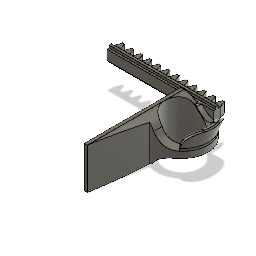
920-002_DynamicFinger (Autodesk Fusion 360 design; units mm, degrees)
Autodesk Fusion 360 part; units mm, degrees
sketch "Sketch1" plane through (0, 0, 0) normal (0, 1, 0) x (1, 0, 0)
  line L0 (0, 0) -> (-12, 0) construction
  line L1 (0.72794, -2) -> (-0.72794, 2)
  line L2 (-1.374447, -2) -> (-1.374447, 4.5) construction
  line L3 (-3.476834, -2) -> (-2.020953, 2)
  line L4 (-2.020953, 2) -> (-0.72794, 2)
  line L5 (0.72794, -2) -> (0.72794, -6)
  line L6 (0.72794, -6) -> (-63.952493, -6)
  line L7 (-4.769847, -2) -> (-6.225728, 2)
  line L8 (-7.51874, 2) -> (-6.225728, 2)
  line L9 (-8.974621, -2) -> (-7.51874, 2)
  line L10 (-10.267634, -2) -> (-11.723515, 2)
  line L11 (-13.016527, 2) -> (-11.723515, 2)
  line L12 (-14.472408, -2) -> (-13.016527, 2)
  line L13 (-15.765421, -2) -> (-17.221302, 2)
  line L14 (-18.514315, 2) -> (-17.221302, 2)
  line L15 (-19.970195, -2) -> (-18.514315, 2)
  line L16 (-21.263208, -2) -> (-22.719089, 2)
  line L17 (-24.012102, 2) -> (-22.719089, 2)
  line L18 (-25.467983, -2) -> (-24.012102, 2)
  line L19 (-26.760995, -2) -> (-28.216876, 2)
  line L20 (-29.509889, 2) -> (-28.216876, 2)
  line L21 (-30.96577, -2) -> (-29.509889, 2)
  line L22 (-32.258782, -2) -> (-33.714663, 2)
  line L23 (-35.007676, 2) -> (-33.714663, 2)
  line L24 (-36.463557, -2) -> (-35.007676, 2)
  line L25 (-37.75657, -2) -> (-39.21245, 2)
  line L26 (-40.505463, 2) -> (-39.21245, 2)
  line L27 (-41.961344, -2) -> (-40.505463, 2)
  line L28 (-43.254357, -2) -> (-44.710238, 2)
  line L29 (-46.00325, 2) -> (-44.710238, 2)
  line L30 (-47.459131, -2) -> (-46.00325, 2)
  line L31 (-48.752144, -2) -> (-50.208025, 2)
  line L32 (-51.501037, 2) -> (-50.208025, 2)
  line L33 (-52.956918, -2) -> (-51.501037, 2)
  line L34 (-54.249931, -2) -> (-55.705812, 2)
  line L35 (-56.998825, 2) -> (-55.705812, 2)
  line L36 (-58.454705, -2) -> (-56.998825, 2)
  line L37 (-59.747718, -2) -> (-61.203599, 2)
  line L38 (-62.496612, 2) -> (-61.203599, 2)
  line L39 (-63.952493, -2) -> (-62.496612, 2)
  line L40 (-63.952493, -2) -> (-63.952493, -6)
  line L41 (-59.747718, -2) -> (-58.454705, -2)
  line L42 (-54.249931, -2) -> (-52.956918, -2)
  line L43 (-48.752144, -2) -> (-47.459131, -2)
  line L44 (-43.254357, -2) -> (-41.961344, -2)
  line L45 (-37.75657, -2) -> (-36.463557, -2)
  line L46 (-32.258782, -2) -> (-30.96577, -2)
  line L47 (-26.760995, -2) -> (-25.467983, -2)
  line L48 (-21.263208, -2) -> (-19.970195, -2)
  line L49 (-15.765421, -2) -> (-14.472408, -2)
  line L50 (0.72794, -2) -> (-4.769847, -2) construction
  line L51 (-8.974621, -2) -> (-10.267634, -2) construction
  line L52 (-10.267634, -2) -> (-8.974621, -2)
  line L53 (-4.769847, -2) -> (-3.476834, -2)
  point P0 (-2.748894, 0)
  dimension "d3" = 70
  dimension "d4" = 2.748894
  dimension "d5" = 2
  dimension "d8" = -5.497787
  dimension "d9" = 0
  dimension "d10" = 4
  constraint coincident L0.start origin
  constraint horizontal L0
  constraint horizontal L50
  constraint midpoint L0.start L1
  constraint perpendicular L2 L50
  constraint perpendicular L5 L50
  constraint perpendicular L5 L6
  constraint vertical L40
  constraint collinear L41 L42
  constraint collinear L42 L43
  constraint collinear L43 L44
  constraint collinear L44 L45
  constraint collinear L45 L46
  constraint collinear L46 L47
  constraint collinear L47 L48
  constraint collinear L48 L49
  constraint collinear L49 L52
  constraint collinear L50 L51
  constraint collinear L52 L53
  measures "d3" angle of L1 L50
  measures "d5" distance of L0 L4
extrude "Extrude1" add sketch "Sketch1" along normal blind 6 contours L1 L3 L4 L5 L6 L7 L8 L9 L10 L11 L12 L13 L14 L15 L16 L17 L18 L19 L20 L21 L22 L23 L24 L25 L26 L27 L28 L29 L30 L31 L32 L33 L34 L35 L36 L37 L38 L39 L40 L41 L42 L43 L44 L45 L46 L47 L48 L49 L52 L53 picked at (-31.827778, -4.666667)
sketch "Sketch3" plane through (0.72794, 0, 0) normal (1, 0, 0) x (0, 0, -1)
  line L0 (-6, 0) -> (-2, 0)
  line L1 (-2, 0) -> (-2, 6)
  line L2 (-2, 6) -> (-6, 6)
  line L3 (-6, 6) -> (-6, 0)
  line L4 (-4.75, 6) -> (-4.75, 7.5)
  line L5 (-4.75, 7.5) -> (-3.25, 7.5)
  line L6 (-3.25, 7.5) -> (-3.25, 6)
  line L7 (-4, 6) -> (-4, 0) construction
  line L8 (-4, 6) -> (-4, 7.5) construction
  line L9 (-4, 3) -> (-2.683417, 3) construction
  line L10 (-4.75, 0) -> (-4.75, -1.5)
  line L11 (-4.75, -1.5) -> (-3.25, -1.5)
  line L12 (-3.25, -1.5) -> (-3.25, 0)
  dimension "d15" = 1.5
  dimension "d16" = 1.5
  constraint coincident L2 L4.start
  constraint perpendicular L2 L4
  constraint perpendicular L4 L5
  constraint coincident L2 L6.end
  constraint midpoint L2 L7.start
  constraint midpoint L0 L7.end
  constraint midpoint L5 L8.end
  constraint vertical L8
  constraint vertical L6
  constraint midpoint L7 L9.start
  constraint perpendicular L7 L9
  constraint symmetric L4.start L9 L10.start
  constraint symmetric L4.end L9 L10.end
  constraint symmetric L5.end L9 L11.end
  constraint symmetric L6.end L9 L12.end
  measures "d15" distance of L4.end L5.end
  measures "d16" distance of L4.start L4.end
extrude "Extrude3" add sketch "Sketch3" against normal blind 64.68 contours L0 L10 L11 L12 | L2 L4 L5 L6 picked at (-3.75, -1) picked at (-3.75, 7)
ref_plane "WorkPlane1" through (-18.27206, 3, 4) normal (1, 0, 0) x (0, 0, -1)
ref_plane "WorkPlane2" through (-31.612276, -3.257, 2) normal (0, -1, 0) x (-1, 0, 0)
sketch "Sketch4" plane through (0, 0, 6) normal (0, 0, 1) x (1, 0, 0)
  line L0 (-63.952493, 0) -> (0.72794, 0)
  line L1 (0.72794, 0) -> (0.72794, 6)
  line L2 (0.72794, 6) -> (-63.952493, 6)
  line L3 (-63.952493, 6) -> (-63.952493, 0)
  line L4 (7.195984, -3.257) -> (-70.420536, -3.257) construction
  line L5 (-18.27206, 24.190027) -> (-18.27206, -18.190027) construction
  line L6 (-18.27206, 9.243) -> (-16.27206, 9.243)
  line L7 (-16.27206, 9.243) -> (-16.27206, -15.757)
  line L8 (-16.27206, -15.757) -> (-18.27206, -15.757)
  line L9 (-18.27206, -15.757) -> (-18.27206, 9.243)
  line L10 (-18.27206, 9.243) -> (-16.27206, -15.757) construction
  line L11 (-16.27206, 9.243) -> (-18.27206, -15.757) construction
  point P0 (-17.27206, -3.257)
  dimension "d21" = 25
  dimension "d22" = 2
  constraint perpendicular L6 L7
  constraint parallel L6 L8
  constraint parallel L7 L9
  constraint horizontal L6
extrude "Extrude4" add sketch "Sketch4" along normal blind 59.5 contours L0 L2 L7 L9 | L0 L7 L8 L9 | L2 L6 L7 L9 picked at (-16.938726, 4) picked at (-16.938726, -10.504667) picked at (-17.605393, 8.162)
sketch "Sketch5" plane through (0, 9.243, 0) normal (0, 1, 0) x (-1, 0, 0)
  line L0 (16.27206, 6) -> (18.27206, 6)
  line L1 (18.27206, 6) -> (18.27206, 65.5)
  line L2 (18.27206, 65.5) -> (16.27206, 65.5)
  line L3 (16.27206, 65.5) -> (16.27206, 6)
  line L4 (-0.72794, 6) -> (16.27206, 6)
  line L5 (16.27206, 65.5) -> (6.27206, 6)
  line L6 (6.27206, 6) -> (16.27206, 6)
  line L7 (16.27206, 6) -> (16.27206, 65.5)
  dimension "d25" = 10
extrude "Extrude5" add sketch "Sketch5" against normal blind 25 contours L3 L4 L5 L6 L7 picked at (12.938726, 25.833333)
sketch "Sketch6" plane through (0, 9.243, 0) normal (0, 1, 0) x (-1, 0, 0)
  line L0 (6.27206, 6) -> (18.27206, 6)
  line L1 (18.27206, 6) -> (18.27206, 65.5)
  line L2 (18.27206, 65.5) -> (16.27206, 65.5)
  line L3 (16.27206, 65.5) -> (6.27206, 6)
  line L4 (16.27206, 65.5) -> (16.27206, -17.848583) construction
  circle A0 centre (5.77206, 18.5) radius 10.5
  circle A1 centre (5.77206, 18.5) radius 15.5
  line L5 (5.77206, 18.5) -> (5.77206, 8) construction
  line L6 (6.27206, 6) -> (-0.72794, 6)
  line L7 (16.27206, 65.5) -> (6.27206, 6)
  line L8 (-0.72794, 6) -> (-0.72794, 4.75)
  line L9 (-0.72794, 4.75) -> (-0.72794, 3.25)
  line L10 (-0.72794, 6) -> (6.27206, 6)
  dimension "d28" = 21
  dimension "d29" = 5
  dimension "d30" = 2
  constraint perpendicular L0 L4
  constraint tangent L4 A0
  measures "d28" diameter of A0
extrude "Extrude6" add sketch "Sketch6" against normal blind 25 contours L3 A0 A1 L6 L7 L8 L9 L10 picked at (-1.91992, 7.664105)
sketch "Sketch7" plane through (0, 9.243, 0) normal (0, 1, 0) x (-1, 0, 0)
  line L0 (9.989032, 28.115984) -> (6.613875, 8.0338)
  arc A0 (9.989032, 28.115984) -> (6.613875, 8.0338) centre (5.77206, 18.5) ccw
  arc A1 (10.835048, 33.149783) -> (-0.72794, 4.428753) centre (5.77206, 18.5) ccw
  line L1 (-0.72794, 4.428753) -> (-0.72794, 6)
  line L2 (-0.72794, 6) -> (18.27206, 6)
  line L3 (18.27206, 6) -> (18.27206, 65.5)
  line L4 (18.27206, 65.5) -> (16.27206, 65.5)
  line L5 (16.27206, 65.5) -> (10.835048, 33.149783)
  circle A2 centre (5.77206, 18.5) radius 10.5
  line L6 (-0.72794, 6) -> (-3.393092, 6)
  constraint concentric A0 A2
  constraint perpendicular L1 L6
extrude "Extrude7" cut sketch "Sketch7" against normal through all contours L0 A2 | A1 L1 L6 picked at (9.219892, 15.192215) picked at (-1.035493, 5.107205)
sketch "Sketch8" plane through (0, 0, 0) normal (0, -1, 0) x (1, 0, 0)
  line L0 (-63.95206, 4.75) -> (0.72794, 4.75)
  line L1 (0.72794, 4.75) -> (0.72794, 6)
  line L2 (0.72794, 6) -> (-18.27206, 6)
  line L3 (-18.27206, 6) -> (-63.952493, 6)
  line L4 (-63.952493, 6) -> (-63.952493, 2)
  line L5 (-63.952493, 2) -> (-62.496612, -2)
  line L6 (-62.496612, -2) -> (-61.203599, -2)
  line L7 (-61.203599, -2) -> (-59.747718, 2)
  line L8 (-59.747718, 2) -> (-58.454705, 2)
  line L9 (-58.454705, 2) -> (-56.998825, -2)
  line L10 (-56.998825, -2) -> (-55.705812, -2)
  line L11 (-55.705812, -2) -> (-54.249931, 2)
  line L12 (-54.249931, 2) -> (-52.956918, 2)
  line L13 (-52.956918, 2) -> (-51.501037, -2)
  line L14 (-51.501037, -2) -> (-50.208025, -2)
  line L15 (-50.208025, -2) -> (-48.752144, 2)
  line L16 (-48.752144, 2) -> (-47.459131, 2)
  line L17 (-47.459131, 2) -> (-46.00325, -2)
  line L18 (-46.00325, -2) -> (-44.710238, -2)
  line L19 (-44.710238, -2) -> (-43.254357, 2)
  line L20 (-43.254357, 2) -> (-41.961344, 2)
  line L21 (-41.961344, 2) -> (-40.505463, -2)
  line L22 (-40.505463, -2) -> (-39.21245, -2)
  line L23 (-39.21245, -2) -> (-37.75657, 2)
  line L24 (-37.75657, 2) -> (-36.463557, 2)
  line L25 (-36.463557, 2) -> (-35.007676, -2)
  line L26 (-35.007676, -2) -> (-33.714663, -2)
  line L27 (-33.714663, -2) -> (-32.258782, 2)
  line L28 (-32.258782, 2) -> (-30.96577, 2)
  line L29 (-30.96577, 2) -> (-29.509889, -2)
  line L30 (-29.509889, -2) -> (-28.216876, -2)
  line L31 (-28.216876, -2) -> (-26.760995, 2)
  line L32 (-26.760995, 2) -> (-25.467983, 2)
  line L33 (-25.467983, 2) -> (-24.012102, -2)
  line L34 (-24.012102, -2) -> (-22.719089, -2)
  line L35 (-22.719089, -2) -> (-21.263208, 2)
  line L36 (-21.263208, 2) -> (-19.970195, 2)
  line L37 (-19.970195, 2) -> (-18.514315, -2)
  line L38 (-18.514315, -2) -> (-17.221302, -2)
  line L39 (-17.221302, -2) -> (-15.765421, 2)
  line L40 (-15.765421, 2) -> (-14.472408, 2)
  line L41 (-14.472408, 2) -> (-13.016527, -2)
  line L42 (-13.016527, -2) -> (-11.723515, -2)
  line L43 (-11.723515, -2) -> (-10.267634, 2)
  line L44 (-10.267634, 2) -> (-8.974621, 2)
  line L45 (-8.974621, 2) -> (-7.51874, -2)
  line L46 (-7.51874, -2) -> (-6.225728, -2)
  line L47 (-6.225728, -2) -> (-4.769847, 2)
  line L48 (-4.769847, 2) -> (-3.476834, 2)
  line L49 (-3.476834, 2) -> (-2.020953, -2)
  line L50 (-2.020953, -2) -> (-0.72794, -2)
  line L51 (-0.72794, -2) -> (0.72794, 2)
  line L52 (0.72794, 2) -> (0.72794, 3.25)
  line L53 (0.72794, 3.25) -> (-63.95206, 3.25)
  line L54 (-63.95206, 3.25) -> (-63.95206, 4.75)
  arc A0 (3.393092, 6) -> (-10.835048, 33.149783) centre (-5.77206, 18.5) ccw
  line L55 (0.72794, 2) -> (0.72794, 3.25)
  line L56 (0.72794, 4.75) -> (0.72794, 3.25)
  line L57 (0.72794, 4.75) -> (0.72794, 6)
  circle A1 centre (-5.77206, 18.5) radius 15.5
  line L58 (3.393092, 6) -> (-18.27206, 6)
  constraint concentric A0 A1
extrude "Extrude8" add sketch "Sketch8" against normal blind 6 contours L1 L56 L57 A1 L58 picked at (1.639612, 5.436751)
sketch "Sketch9" plane through (0, 0, 6) normal (0, 0, 1) x (1, 0, 0)
  line L0 (-18.27206, 0) -> (-18.27206, 6)
  line L1 (-18.27206, 6) -> (-63.952493, 6)
  line L2 (-63.952493, 6) -> (-63.952493, 0)
  line L3 (-63.952493, 0) -> (-18.27206, 0)
  line L4 (-16.27206, -15.757) -> (-16.27206, 9.243)
  line L5 (-16.27206, -1.318142) -> (-5.710918, -1.318142) construction
  line L6 (-16.27206, -5.195858) -> (-5.710918, -5.195858) construction
  line L7 (-5.710918, -1.318142) -> (-5.710918, -5.195858) construction
  arc A0 (-5.710918, -1.318142) -> (-16.27206, 9.243) centre (-16.27206, -1.318142) ccw
  arc A1 (-16.27206, 5.365283) -> (-18.27206, 5.174181) centre (-16.27206, -5.195858) ccw
  arc A2 (-16.27206, -15.757) -> (-5.710918, -5.195858) centre (-16.27206, -5.195858) ccw
  line L8 (9.72794, 9.243) -> (-10.835048, 9.243)
  line L9 (-10.835048, -15.757) -> (9.72794, -15.757)
  line L10 (9.72794, 9.243) -> (9.72794, -15.757)
  line L11 (-16.27206, 9.243) -> (9.72794, 9.243)
  line L12 (-16.27206, -15.757) -> (9.72794, -15.757)
  line L13 (-5.710918, -1.318142) -> (9.72794, -1.318142)
  line L14 (-5.710918, -5.195858) -> (9.72794, -5.195858)
  point P0 (-16.27206, 9.243)
  dimension "d36" = 21.122283
  constraint equal A0 A1
  constraint perpendicular L4 L5
  constraint perpendicular L4 L6
  constraint concentric A1 A2
  constraint perpendicular L10 L13
  constraint perpendicular L10 L14
  measures "d36" diameter of A0
extrude "Extrude9" cut sketch "Sketch9" along normal through all contours A2 L9 L10 L12 L14 | A0 L8 L10 L11 L13 picked at (4.439054, -9.708045) picked at (4.439054, 3.194045)
fillet "Fillet1" radius 15 4 edges at (-5.710918, -1.318142, 7.000089) (-5.710918, -1.318142, 31.499851) (-5.710918, -5.195858, 31.499851) (-5.710918, -5.195858, 7.000089)
sketch "Sketch10" plane through (0, 6, 0) normal (0, 1, 0) x (-1, 0, 0)
  line L0 (63.95206, 3.25) -> (-0.72794, 3.25)
  line L1 (-0.72794, 3.25) -> (-0.72794, 2)
  line L2 (-0.72794, 2) -> (0.72794, -2)
  line L3 (0.72794, -2) -> (2.020953, -2)
  line L4 (2.020953, -2) -> (3.476834, 2)
  line L5 (3.476834, 2) -> (4.769847, 2)
  line L6 (4.769847, 2) -> (6.225728, -2)
  line L7 (6.225728, -2) -> (7.51874, -2)
  line L8 (7.51874, -2) -> (8.974621, 2)
  line L9 (8.974621, 2) -> (10.267634, 2)
  line L10 (10.267634, 2) -> (11.723515, -2)
  line L11 (11.723515, -2) -> (13.016527, -2)
  line L12 (13.016527, -2) -> (14.472408, 2)
  line L13 (14.472408, 2) -> (15.765421, 2)
  line L14 (15.765421, 2) -> (17.221302, -2)
  line L15 (17.221302, -2) -> (18.514315, -2)
  line L16 (18.514315, -2) -> (19.970195, 2)
  line L17 (19.970195, 2) -> (21.263208, 2)
  line L18 (21.263208, 2) -> (22.719089, -2)
  line L19 (22.719089, -2) -> (24.012102, -2)
  line L20 (24.012102, -2) -> (25.467983, 2)
  line L21 (25.467983, 2) -> (26.760995, 2)
  line L22 (26.760995, 2) -> (28.216876, -2)
  line L23 (28.216876, -2) -> (29.509889, -2)
  line L24 (29.509889, -2) -> (30.96577, 2)
  line L25 (30.96577, 2) -> (32.258782, 2)
  line L26 (32.258782, 2) -> (33.714663, -2)
  line L27 (33.714663, -2) -> (35.007676, -2)
  line L28 (35.007676, -2) -> (36.463557, 2)
  line L29 (36.463557, 2) -> (37.75657, 2)
  line L30 (37.75657, 2) -> (39.21245, -2)
  line L31 (39.21245, -2) -> (40.505463, -2)
  line L32 (40.505463, -2) -> (41.961344, 2)
  line L33 (41.961344, 2) -> (43.254357, 2)
  line L34 (43.254357, 2) -> (44.710238, -2)
  line L35 (44.710238, -2) -> (46.00325, -2)
  line L36 (46.00325, -2) -> (47.459131, 2)
  line L37 (47.459131, 2) -> (48.752144, 2)
  line L38 (48.752144, 2) -> (50.208025, -2)
  line L39 (50.208025, -2) -> (51.501037, -2)
  line L40 (51.501037, -2) -> (52.956918, 2)
  line L41 (52.956918, 2) -> (54.249931, 2)
  line L42 (54.249931, 2) -> (55.705812, -2)
  line L43 (55.705812, -2) -> (56.998825, -2)
  line L44 (56.998825, -2) -> (58.454705, 2)
  line L45 (58.454705, 2) -> (59.747718, 2)
  line L46 (59.747718, 2) -> (61.203599, -2)
  line L47 (61.203599, -2) -> (62.496612, -2)
  line L48 (62.496612, -2) -> (63.952493, 2)
  line L49 (63.952493, 2) -> (63.952493, 6)
  line L50 (63.952493, 6) -> (18.27206, 6)
  line L51 (18.27206, 6) -> (8.657434, 6)
  line L52 (8.657434, 6) -> (-3.393092, 6)
  arc A0 (-3.393092, 6) -> (-0.72794, 4.428753) centre (5.77206, 18.5) ccw
  line L53 (-0.72794, 4.428753) -> (-0.72794, 4.75)
  line L54 (-0.72794, 4.75) -> (63.95206, 4.75)
  line L55 (63.95206, 4.75) -> (63.95206, 3.25)
  line L56 (-0.72794, 4.428753) -> (-0.72794, 6)
  constraint vertical L56
extrude "Extrude10" cut sketch "Sketch10" against normal blind 7 contours L52 A0 L53 L56 picked at (-1.639612, 5.436751)
chamfer "Chamfer1" distance 1.8 angle 45 2 edges at (-8.169613, 5.455932, 6) (-5.041875, 2.046714, 6)
sketch "Sketch11" plane through (-18.27206, 0, 0) normal (-1, 0, 0) x (0, 0, 1)
  line L0 (6, 0) -> (6, -15.757) construction
  line L1 (6, -15.757) -> (65.5, -15.757) construction
  line L2 (65.5, -15.757) -> (65.5, 9.243) construction
  line L3 (65.5, 9.243) -> (6, 9.243) construction
  line L4 (6, 9.243) -> (6, 6) construction
  line L5 (6, 6) -> (6, 0) construction
  line L6 (8.634048, 5.743) -> (8.634048, -0.257) construction
  line L7 (8.634048, -0.257) -> (8.634048, -13.257) construction
  line L8 (8.634048, -13.257) -> (63.134048, -13.257) construction
  line L9 (63, -13.514) -> (63, 6.743) construction
  line L10 (63, 6.743) -> (8.634048, 6.743) construction
  line L11 (8.634048, 6.743) -> (8.634048, 5.743) construction
  line L12 (51.5, 1.743) -> (51.5, -8.257)
  arc A0 (61.5, 1.743) -> (51.5, 1.743) centre (56.5, 1.743) ccw
  line L13 (41.5, 1.743) -> (41.5, -8.257)
  arc A1 (41.5, -8.257) -> (51.5, -8.257) centre (46.5, -8.257) ccw
  line L14 (51.5, 1.743) -> (41.5, 1.743) construction
  line L15 (61.5, 1.743) -> (61.5, -13.257)
  line L16 (21.5, 1.743) -> (21.5, -8.257)
  arc A2 (21.5, -8.257) -> (31.5, -8.257) centre (26.5, -8.257) ccw
  line L17 (31.5, 1.743) -> (31.5, -8.257)
  arc A3 (41.5, 1.743) -> (31.5, 1.743) centre (36.5, 1.743) ccw
  line L18 (1.5, 1.743) -> (1.5, -8.257) construction
  arc A4 (1.5, -8.257) -> (11.5, -8.257) centre (6.5, -8.257) ccw construction
  line L19 (11.5, 1.743) -> (11.5, -8.257)
  arc A5 (21.5, 1.743) -> (11.5, 1.743) centre (16.5, 1.743) ccw
  dimension "d43" = 10
  dimension "d44" = 10
  dimension "d51" = 1.5
  dimension "d52" = 2.5
  dimension "d53" = 2.5
  dimension "d54" = 2.5
  dimension "d57" = -20
  dimension "d58" = 0
  constraint perpendicular L8 L12
  constraint tangent L12 A0
  constraint tangent L10 A0
  constraint tangent L12 A1
  constraint tangent L8 A1
  constraint perpendicular L10 L13
  constraint tangent L13 A1
  constraint perpendicular L13 L14
  constraint parallel L5 L6
  constraint parallel L0 L7
  constraint parallel L1 L8
  constraint parallel L2 L9
  constraint parallel L3 L10
  constraint parallel L4 L11
  constraint coincident L8 L15.end
  constraint tangent A0 L15
  constraint vertical L15
  measures "d43" diameter of A0
  measures "d44" diameter of A1
  measures "d51" distance of L9 L15
  measures "d52" distance of L2 L9
  measures "d53" distance of L3 L10
  measures "d54" distance of L1 L8
ref_plane "WorkPlane3" through (-17.27206, -13.257, 35.75) normal (0, -1, 0) x (1, 0, 0)
sketch "Sketch12" plane through (-17.27206, -13.257, 35.75) normal (0, -1, 0) x (1, 0, 0)
  circle A0 centre (-1, 25.75) radius 1 construction
  line L0 (-1, 26.75) -> (-0.6, 26.75)
  line L1 (-0.6, 26.75) -> (0.4, 27.75)
  line L2 (0.4, 27.75) -> (0.4, 23.75)
  line L3 (0.4, 23.75) -> (-0.6, 24.75)
  line L4 (-0.6, 24.75) -> (-1, 24.75)
  line L5 (-1, 26.75) -> (-1, 24.75)
  point P0 (-1, 25.75)
  dimension "d46" = 2
  dimension "d47" = 45
  dimension "d48" = 45
  dimension "d49" = 0.4
  dimension "d50" = 1
  constraint coincident P0 A0.centre
  constraint coincident A0 L0.start
  constraint tangent A0 L0
  constraint perpendicular L0 L2
  constraint coincident A0 L4.end
  constraint horizontal L4
  constraint vertical L2
  constraint equal L0 L4
  constraint vertical L5
  measures "d46" diameter of A0
  measures "d47" angle of L1 L2
  measures "d48" angle of L2 L3
  measures "d49" distance of L3.end L4.end
  measures "d50" distance of L2 L3.end
sweep "Sweep1" [suppressed]
extrude "Extrude11" cut 2 faces at (-8.224318, -2.75777, 6) (-17.605393, 8.162, 6) along direction (0, 0, 1) blind 1
extrude "Extrude12" cut 1 faces at (3.393092, -2.598866, 6.333333) along direction (1, 0, 0) blind 17
chamfer "Chamfer3" distance 1 angle 45 2 edges at (-13.464747, 6, 7) (-9.997845, 0, 7)
sketch "Sketch13" plane through (-18.27206, 0, 0) normal (-1, 0, 0) x (0, 0, 1)
  line L0 (7, -1) -> (7, -15.757)
  line L1 (7, -15.757) -> (65.5, -15.757)
  line L2 (65.5, -15.757) -> (65.5, 9.243)
  line L3 (65.5, 9.243) -> (7, 9.243)
  line L4 (7, 9.243) -> (7, 7)
  line L5 (7, 7) -> (6, 6)
  line L6 (6, 6) -> (6, 0)
  line L7 (6, 0) -> (7, -1)
  line L8 (63, 6.743) -> (13, 6.743)
  line L9 (13, 6.743) -> (13, -13.257)
  line L10 (13, -13.257) -> (63, -13.257)
  line L11 (63, -13.257) -> (63, 6.743)
  dimension "d72" = 2.5
  dimension "d73" = 2.5
  dimension "d74" = 2.5
  dimension "d75" = 50
  constraint horizontal L8
  constraint vertical L9
  constraint horizontal L10
  constraint vertical L11
  measures "d72" distance of L2 L11
  measures "d73" distance of L3 L8
  measures "d74" distance of L1 L10
  measures "d75" distance of L8.start L8.end
extrude "Extrude13" [suppressed]
ref_plane "WorkPlane4" through (-5.77206, -3.251022, 18.5) normal (0, 0, 1) x (0, -1, 0)
sketch "Sketch14" plane through (-5.77206, -3.251022, 18.5) normal (0, 0, 1) x (1, 0, 0)
  line L0 (10.5, 1.932881) -> (10.197149, 1.932881)
  line L1 (10.5, 1.932881) -> (10.5, -2.146312)
  line L2 (10.5, 1.932881) -> (25.341899, 1.932881) construction
  line L3 (10.197149, 1.932881) -> (15.5, 1.932881)
  line L4 (11.169873, 4.432881) -> (15.823975, 12.494022)
  line L5 (16.573975, 13.793061) -> (18.823975, 12.494022)
  line L6 (18.823975, 12.494022) -> (15.768443, 3.549164)
  arc A0 (11.169873, 4.432881) -> (10.5, 1.932881) centre (15.5, 1.932881) ccw
  arc A1 (15.768443, 3.549164) -> (15.5, 1.932881) centre (20.5, 1.932881) ccw
  line L7 (-10.5, 12.494022) -> (-12.5, 12.494022) construction
  line L8 (18.823975, 12.494022) -> (15.823975, 12.494022)
  dimension "d80" = 10
  dimension "d99" = 60
  dimension "d100" = 3
  constraint perpendicular L0 L1
  constraint tangent L1 A0
  constraint perpendicular L1 L2
  constraint equal A0 A1
  constraint perpendicular L4 L5
  constraint tangent L6 A1
  constraint tangent L4 A0
  constraint horizontal L8
  measures "d80" diameter of A1
  measures "d99" angle of L2 L4
revolve "Revolve1" add sketch "Sketch14" angle 50 about axis through (-5.77206, 21.751506, 18.5) along (0, -1, 0) second angle 50 contours L3 L4 L6 A0 A1 L8 picked at (14.254097, 6.825356)
ref_plane "WorkPlane5" through (20, 0, 0) normal (1, 0, 0) x (0, 1, 0)
ref_plane "WorkPlane6" through (-5.77206, -3.251022, 18.5) normal (0.642788, 0, 0.766044) x (0, -1, 0)
sketch "Sketch16" plane through (-5.77206, -3.251022, 18.5) normal (0.642788, 0, 0.766044) x (0, -1, 0)
  line L0 (-1.932881, 0.307955) -> (-1.932881, 15.5)
  spline S0 degree 3 poles (-8.130457, -11.376824) (-7.72598, -11.175944) (-7.336663, -10.956348) (-6.061278, -10.135244) (-5.262841, -9.436609) (-3.927766, -7.822272) (-3.336234, -6.826048) (-2.480713, -4.618506) (-2.213766, -3.40663) (-1.987199, -1.51225) (-1.943763, -0.758068) (-1.934705, 0) knots 5.34591585 5.34591585 5.34591585 5.34591585 5.49176143 5.49176143 5.84658734 5.84658734 6.19902731 6.19902731 6.55146729 6.55146729 6.77744579 6.77744579 6.77744579 6.77744579
  line L1 (-14.659086, 0) -> (-1.934705, 0)
  line L2 (-14.659086, 12.726205) -> (-14.659086, 0)
  circle A0 centre (-1.932881, 10.561142) radius 10.561142
  line L3 (-12.494022, 0) -> (-12.494022, 18.823975)
  line L4 (-12.494022, 0) -> (-1.934705, 0)
  constraint tangent L1 A0
  constraint tangent A0 L3
extrude "Extrude16" cut sketch "Sketch16" along normal through all contours L1 A0 L3 L4 picked at (-10.419578, 2.075302)
ref_plane "WorkPlane7" through (-5.77206, -3.251022, 18.5) normal (-0.642788, 0, 0.766044) x (0, -1, 0)
sketch "Sketch18" plane through (0, -1.318142, 0) normal (0, -1, 0) x (1, 0, 0)
  line L0 (4.620245, 7) -> (3.877586, 7)
  line L1 (3.877586, 7) -> (4.191148, 6.626311)
  arc A0 (4.191148, 6.626311) -> (4.620245, 7) centre (-5.77206, 18.5) ccw construction
  line L2 (3.877586, 7) -> (9.130693, 7)
  line L3 (6.327759, 4.079998) -> (4.3637, 6.420672)
  arc A1 (6.327759, 4.079998) -> (12.334277, 23.648071) centre (-5.77206, 18.5) ccw
  line L4 (3.877586, 7) -> (6.327759, 4.079998)
  constraint parallel L0 L2
extrude "Extrude19" cut sketch "Sketch18" against normal through all contours L0 L1 L2 L3 A1 L4 picked at (6.007561, 5.162004)
sketch "Sketch17" plane through (-5.77206, -3.251022, 18.5) normal (-0.642788, 0, 0.766044) x (0, -1, 0)
  line L0 (-12.494022, 4.024114) -> (-12.494022, 17.179375)
  circle A0 centre (-1.932881, 10.561142) radius 10.561142
  line L1 (-12.494022, 10.561142) -> (-12.494022, 4.024114)
  line L2 (-1.932881, 0.56891) -> (-1.932881, 15.5)
  line L3 (-12.494022, 10.561142) -> (-12.494022, 0)
  line L4 (-11.087958, 0) -> (-1.942876, 0)
  line L5 (-12.494022, 0) -> (-1.942876, 0)
  constraint tangent L0 A0
  constraint tangent A0 L1
  constraint tangent A0 L4
  constraint vertical L3
  constraint tangent A0 L5
extrude "Extrude20" cut sketch "Sketch17" against normal blind 36 contours L0 A0 L1 L3 L4 L5 picked at (-11.166471, 2.557538)
fillet "Fillet2" radius 3 5 edges at (1.203835, 0.171882, 26.649181) (6.357749, 7.049053, 26.548039) (10.051916, 9.243, 18.5) (6.357749, 7.049053, 10.451961) (1.203836, 0.171885, 10.350818)
sketch "Sketch19" plane through (0, 0, 65.5) normal (0, 0, 1) x (1, 0, 0)
  line L0 (-18.27206, -15.757) -> (-16.27206, -15.757)
  line L1 (-16.27206, -15.757) -> (-16.27206, 9.243)
  line L2 (-16.27206, 9.243) -> (-18.27206, 9.243)
  line L3 (-18.27206, 9.243) -> (-18.27206, -15.757)
  spline S0 degree 3 poles (-20.741363, -3.646192) (-20.740312, -4.532238) (-20.536724, -5.296386) (-20.0708, -6.621522) (-19.772716, -7.229425) (-19.467056, -8.742265) (-19.500976, -9.359009) (-19.690881, -10.459329) (-19.920787, -11.070973) (-20.87865, -12.564312) (-21.671721, -13.081104) (-22.883396, -13.987902) (-23.425332, -14.422225) (-24.525015, -15.849757) (-24.834803, -16.655796) (-25.232434, -18.140954) (-25.297764, -18.85444) (-25.727447, -20.040821) (-25.982198, -20.620265) (-26.909383, -21.691182) (-27.418557, -22.094346) (-28.868485, -22.813385) (-29.702348, -22.903075) (-30.398889, -22.947423) (-31.254391, -23.001891) (-32.293925, -23.026249) (-34.515115, -23.984995) (-35.255246, -24.70291) (-36.266794, -25.737962) (-36.697115, -26.19792) (-37.958104, -26.994139) (-38.566926, -27.181327) (-39.605602, -27.375765) (-40.252299, -27.39354) (-42.031875, -27.012774) (-42.775654, -26.459805) (-44.256636, -25.720546) (-44.918154, -25.442742) (-46.85364, -25.167442) (-47.801701, -25.352066) (-49.176922, -25.666176) (-49.790052, -25.826116) (-51.308682, -25.825518) (-51.92667, -25.648303) (-52.88938, -25.266251) (-53.442984, -24.934012) (-54.68083, -23.724889) (-55.028376, -22.923807) (-55.770572, -21.597014) (-56.139974, -21.002354) (-57.457351, -19.723047) (-58.24792, -19.321118) (-59.628628, -18.767901) (-60.291464, -18.596662) (-61.636765, -17.845387) (-62.083002, -17.424531) (-62.803028, -16.55579) (-63.117997, -15.984345) (-63.669667, -14.157378) (-63.464407, -13.140174) (-63.390349, -11.438434) (-63.402259, -10.727448) (-64.001615, -8.552682) (-64.792746, -7.650317) (-65.698111, -6.423563) (-66.043656, -5.912375) (-66.478916, -4.632957) (-66.570246, -4.010372) (-66.507896, -2.923782) (-66.419864, -2.276829) (-65.63308, -0.656851) (-65.058724, -0.084639) (-64.175977, 1.236791) (-63.816969, 1.87351) (-63.332981, 3.764359) (-63.403565, 4.708729) (-63.519308, 6.088986) (-63.575781, 6.712375) (-63.324119, 8.213592) (-63.038841, 8.798033) (-62.517487, 9.656722) (-62.10243, 10.151784) (-60.746053, 11.139431) (-59.95771, 11.362775) (-58.589381, 11.883243) (-57.94788, 12.158421) (-56.490984, 13.260431) (-55.975188, 13.974411) (-55.213681, 15.271686) (-54.951664, 15.911879) (-54.026922, 17.139143) (-53.558274, 17.525813) (-52.584311, 18.13195) (-51.976644, 18.366718) (-50.108622, 18.665422) (-49.129698, 18.336774) (-47.503093, 18.014899) (-46.804953, 17.915194) (-44.901512, 18.11841) (-44.042596, 18.514123) (-42.764122, 19.208753) (-42.215523, 19.564483) (-40.758823, 20.046232) (-40.129487, 20.077812) (-39.043787, 20.019031) (-38.415174, 19.864502) (-36.89026, 19.127789) (-36.296643, 18.467837) (-35.272086, 17.434766) (-34.771563, 16.955827) (-33.221583, 16.054153) (-32.393278, 15.851592) (-30.85266, 15.647777) (-30.119304, 15.690992) (-28.859034, 15.44009) (-28.250335, 15.274999) (-27.05682, 14.52504) (-26.581678, 14.084065) (-25.443883, 12.469004) (-25.344157, 11.376358) (-24.939112, 9.712713) (-24.732145, 9.034537) (-23.733217, 7.395128) (-23.007882, 6.78684) (-21.855811, 5.92821) (-21.312607, 5.575772) (-20.2811, 4.445193) (-19.995827, 3.879285) (-19.60939, 2.868307) (-19.494742, 2.231365) (-19.549241, 0.46494) (-19.960569, -0.372986) (-20.491157, -1.858239) (-20.694612, -2.530437) (-20.739161, -3.458852) (-20.7413, -3.553193) (-20.741363, -3.646192) knots 2.80887435 2.80887435 2.80887435 2.80887435 3.00198904 3.00198904 3.22215989 3.22215989 3.42641671 3.42641671 3.69168647 3.69168647 4.13096445 4.13096445 4.39699529 4.39699529 4.71403678 4.71403678 5.08002219 5.08002219 5.26312438 5.26312438 5.40836336 5.40836336 5.61774869 5.61774869 5.61774869 5.87491911 5.87491911 6.12013444 6.12013444 6.30224574 6.30224574 6.48452111 6.48452111 6.70441823 6.70441823 7.04510995 7.04510995 7.22773487 7.22773487 7.4616181 7.4616181 7.64892212 7.64892212 7.84103943 7.84103943 8.09229154 8.09229154 8.45740053 8.45740053 8.67732203 8.67732203 8.94365892 8.94365892 9.22421415 9.22421415 9.47865504 9.47865504 9.80004433 9.80004433 10.39844102 10.39844102 10.70399939 10.70399939 11.21208264 11.21208264 11.46666155 11.46666155 11.67689973 11.67689973 11.82234832 11.82234832 11.98205031 11.98205031 12.07623621 12.07623621 12.19168777 12.19168777 12.27805341 12.27805341 12.36914805 12.36914805 12.488352 12.488352 12.64519136 12.64519136 12.74541679 12.74541679 12.86645653 12.86645653 12.99775671 12.99775671 13.11261122 13.11261122 13.25184444 13.25184444 13.50841841 13.50841841 13.64384621 13.64384621 13.81767248 13.81767248 13.97556694 13.97556694 14.13057024 14.13057024 14.34054812 14.34054812 14.66690275 14.66690275 14.87773553 14.87773553 15.12799805 15.12799805 15.43340773 15.43340773 15.58538871 15.58538871 15.70654387 15.70654387 15.947287 15.947287 16.06822563 16.06822563 16.22232012 16.22232012 16.35905748 16.35905748 16.49525248 16.49525248 16.68189284 16.68189284 16.99251578 16.99251578 17.16897051 17.16897051 17.18923959 17.18923959 17.18923959 17.18923959
  line L4 (-69.260025, 8.743178) -> (-69.260025, -16.256822)
  line L5 (-67.260025, 8.743178) -> (-69.260025, 8.743178)
  line L6 (-18.27206, 9.243) -> (-18.27206, -15.757)
  line L7 (-69.260025, -16.256822) -> (-67.260025, -16.256822)
  line L8 (-67.260025, 8.743178) -> (-69.260025, 8.743178)
  line L9 (-16.27206, 9.243) -> (-18.27206, 9.243)
  line L10 (-67.260025, -16.256822) -> (-67.260025, 8.743178)
  line L11 (-67.260025, -16.256822) -> (-67.260025, 8.743178)
  line L12 (-18.27206, 9.243) -> (-24.755195, 9.243)
  line L13 (-18.27206, -15.757) -> (-24.38094, -15.757)
  point P0 (-68.641363, -9.646191)
  constraint perpendicular L6 L12
  constraint perpendicular L6 L13
extrude "Extrude21" [suppressed]
equation "d4 = ( PI * 21 / 24 ) * 1 mm"
equation "d8 = ( -2 * PI * 21 / 24 ) * 1 mm"
equation "d87 = 50.0 deg - 90 deg"
